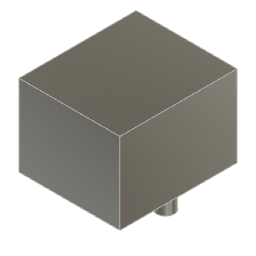
_Ethernet Jack.38e78c15-344b-44d7-bd83-56f5c26b8b03 (Autodesk Fusion 360 design; units mm, degrees)
Autodesk Fusion 360 part; units mm, degrees
sketch "Sketch1" plane through (0, 0, 0) normal (0, 1, 0) x (1, 0, 0)
  line L0 (0, 0) -> (15.5, 0)
  line L1 (15.5, 0) -> (15.5, -12.5)
  line L2 (15.5, -12.5) -> (0, -12.5)
  line L3 (0, -12.5) -> (0, 0)
  line L4 (2, -2) -> (13.5, -2)
  line L5 (13.5, -2) -> (13.5, -10.5)
  line L6 (13.5, -10.5) -> (2, -10.5)
  line L7 (2, -10.5) -> (2, -2)
  dimension "d1" = 15.5
  dimension "d2" = 12.5
  dimension "d3" = 2
  constraint horizontal L0
  constraint vertical L1
  constraint horizontal L2
  constraint vertical L3
  constraint coincident L0.start L3.end
  measures "d1" distance of L0.start L0.end
  measures "d2" distance of L0.start L2.end
extrude "Extrude1" add sketch "Sketch1" along normal blind 18
extrude "Extrude2" add sketch "Sketch1" along normal blind 3 contours L4 L5 L6 L7
sketch "Sketch2" plane through (0, 0, 0) normal (0, 0, -1) x (1, 0, 0)
  line L0 (15.5, 0) -> (0, 0)
  line L1 (0, 0) -> (0, -18)
  line L2 (0, -18) -> (15.5, -18)
  line L3 (15.5, -18) -> (15.5, 0)
  line L4 (0, -18) -> (0, -7)
  line L5 (0, -7) -> (15.5, -7)
  line L6 (15.5, -7) -> (15.5, -18)
  circle A0 centre (14.15, -8.35) radius 1.35
  circle A1 centre (1.35, -8.35) radius 1.35
  dimension "d8" = 11
  dimension "d9" = 1.35
  dimension "d10" = 1.35
  constraint vertical L4
  constraint horizontal L5
  constraint vertical L6
  constraint coincident L2.end L3.start
  constraint tangent L5 A0
  constraint tangent L6 A0
  constraint tangent L5 A1
  constraint tangent L4 A1
  measures "d8" distance of L2.end L5.end
  measures "d9" radius of A0
  measures "d10" radius of A1
extrude "Extrude3" add sketch "Sketch2" along normal blind 2 contours A0 | A1
equation "d9 = ( 2.7 / 2 ) * 1 mm"
equation "d10 = ( 2.7 / 2 ) * 1 mm"
